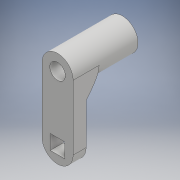
# Autodesk Inventor part: crankshaft_support
Saved by Autodesk Inventor 2018 (Build 220112000, 112)
## iProperties
Created: 2026-05-01
Part Number: crankshaft_support
Material: Generic
Document SubType Name: Modeling
Designer: neo
Density: 1 g/cm^3
Appearance: Default
Author: neo
Autodesk Inventor part; units mm, degrees
ref_plane "YZ Plane" through (0, 0, 0) normal (1, 0, 0) x (0, 1, 0)
ref_plane "XZ Plane" through (0, 0, 0) normal (0, 1, 0) x (-1, 0, 0)
ref_plane "XY Plane" through (0, 0, 0) normal (0, 0, 1) x (1, 0, 0)
sketch "Sketch1" plane through (0, 0, 0) normal (0, 1, 0) x (-1, 0, 0)
  circle A0 centre (0, 0) radius 4 construction
  line L0 (2.8284, 2.8284) -> (-2.8284, 2.8284)
  line L1 (-2.8284, 2.8284) -> (-2.8284, -2.8284)
  line L2 (-2.8284, -2.8284) -> (2.8284, -2.8284)
  line L3 (2.8284, -2.8284) -> (2.8284, 2.8284)
  line L4 (0, 0) -> (0, -10.4382)
  arc A1 (-6, 0) -> (6, 0) centre (0, 0) ccw
  arc A2 (6, 25) -> (-6, 25) centre (0, 25) ccw
  line L5 (6, 25) -> (6, 0)
  line L6 (-6, 25) -> (-6, 0)
  dimension "d0" = 8
  dimension "d1" = 12
  dimension "d2" = 12
  dimension "d5" = 25
  constraints: 14 end point, 7 point on circle, 3 centre point, 3 vertical, 2 coincident, 2 parallel, 2 perpendicular, 1 horizontal
  measures "d0" diameter of A0
  measures "d1" diameter of A1
  measures "d2" diameter of A2
  measures "d5" distance of A1.centre A2.centre
extrude "Extrusion1" add sketch "Sketch1" along normal blind 5
sketch "Sketch2" plane through (0, 5, 0) normal (0, 1, 0) x (1, 0, 0)
  arc A0 (-6, -25) -> (6, -25) centre (0, -25) ccw projected
  circle A1 centre (0, -25) radius 6
  point P0 (0, 0)
  constraints: 1 coincident, 1 horizontal alignment, 2 other
extrude "Extrusion2" add sketch "Sketch2" along normal blind 20
hole "Hole1" at (0, 25, 25) direction (0, -1, 0) diameter 6 end through all
chamfer "Chamfer1" distance 5 angle 45 1 edges at (0, 5, 19)
body "Solid1"
